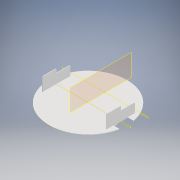
# Autodesk Inventor part: GonjaKonstrukcija_v.1.0
Saved by Autodesk Inventor 2020 (Build 240168000, 168)
## iProperties
Created: 2020-07-10
Part Number: GonjaKonstrukcija_v.1.0
Material: Generic
Document SubType Name: Modeling
Designer: Sičaja
Density: 1 g/cm^3
Appearance: Default
Author: Sičaja
Autodesk Inventor part; units mm, degrees
ref_plane "YZ Plane" through (0, 0, 0) normal (1, 0, 0) x (0, 1, 0)
ref_plane "XZ Plane" through (0, 0, 0) normal (0, 1, 0) x (-1, 0, 0)
ref_plane "XY Plane" through (0, 0, 0) normal (0, 0, 1) x (1, 0, 0)
sketch "Sketch1" plane through (0, 0, 0) normal (0, 1, 0) x (-1, 0, 0)
  circle A0 centre (0, 0) radius 75
  line L0 (20.1131, 19.7531) -> (28.825, 13.0373) projected
  line L1 (28.825, 13.0373) -> (16.004, -3.5946) projected
  line L2 (11.648, -0.2367) -> (16.004, -3.5946) projected
  line L3 (7.292, 3.1212) -> (11.648, -0.2367) projected
  line L4 (20.1131, 19.7531) -> (7.292, 3.1212) projected
  line L5 (4.487, 2.7582) -> (10.4269, -1.8207)
  line L6 (10.4269, -1.8207) -> (16.3669, -6.3997)
  line L7 (16.3669, -6.3997) -> (31.6301, 13.4002)
  line L8 (31.6301, 13.4002) -> (19.7502, 22.5581)
  line L9 (19.7502, 22.5581) -> (4.487, 2.7582)
  line L10 (16.3669, -6.3997) -> (31.6301, 13.4002)
  line L11 (19.7502, 22.5581) -> (4.487, 2.7582)
  line L12 (16.3669, -6.3997) -> (16.004, -3.5946)
  line L13 (28.825, 13.0373) -> (20.1131, 19.7531)
  line L14 (7.292, 3.1212) -> (16.004, -3.5946)
  line L15 (4.487, 2.7582) -> (16.3669, -6.3997)
  line L16 (32.309, 14.2809) -> (20.4291, 23.4389)
  line L17 (20.4291, 23.4389) -> (4.487, 2.7582)
  line L18 (16.3669, -6.3997) -> (32.309, 14.2809)
  line L19 (32.309, 14.2809) -> (16.3669, -6.3997)
  line L20 (4.487, 2.7582) -> (16.3669, -6.3997)
  line L21 (4.487, 2.7582) -> (20.4291, 23.4389)
  line L22 (32.309, 14.2809) -> (16.3669, -6.3997)
  line L23 (0, -32.563) -> (1, -32.563)
  line L24 (1, -32.563) -> (1, -33.063)
  line L25 (1, -33.063) -> (-1, -33.063)
  line L26 (-1, -33.063) -> (-1, -32.563)
  line L27 (-1, -32.563) -> (1, -32.563)
  dimension "d0" = 150
  dimension "d3" = 2
  dimension "d15" = 32.563
  dimension "d16" = 1
  dimension "d18" = 0.5
  dimension "d19" = 2
  dimension "d20" = 0.5
  constraints: 46 end point, 8 perpendicular, 4 collinear, 1 centre point, 1 coincident, 1 parallel, 1 vertical, 4 other
  measures "d0" diameter of A0
  measures "d3" distance between parallel lines of L4 L9
  measures "d15" distance of A0.centre L23.start
  measures "d16" distance of L23.start L23.end
  measures "d18" distance of L23.end L24.end
  measures "d19" distance of L24.end L25.end
  measures "d20" distance of L25.end L26.end
extrude "Extrusion1" add sketch "Sketch1" along normal blind 1 contours A0 | L0 L1 L2 L3 L4 | L9 L8 L7 L6 L5 | L17 L16 L18 L8 | L23 L24 L25 L26 L27
sketch "Sketch2" plane through (0, 0, 0) normal (0, -1, 0) x (1, 0, 0)
  circle A0 centre (0, 0) radius 75 projected
  line L0 (-20.7236, 20.5451) -> (-29.4356, 13.8293) projected
  line L1 (-29.4356, 13.8293) -> (-16.004, -3.5946) projected
  line L2 (-16.004, -3.5946) -> (-7.292, 3.1212) projected
  line L3 (-7.292, 3.1212) -> (-20.7236, 20.5451) projected
  line L4 (-4.487, 2.7582) -> (-16.3669, -6.3997)
  line L5 (-16.3669, -6.3997) -> (-32.2406, 14.1922)
  line L6 (-32.2406, 14.1922) -> (-20.3607, 23.3501)
  line L7 (-20.3607, 23.3501) -> (-4.487, 2.7582)
  dimension "d4" = 2
  constraints: 8 end point, 3 other
  measures "d4" distance between parallel lines of L2 L4
extrude "Extrusion2" cut sketch "Sketch2" against normal blind 1 contours L3 L2 L1 L0 | L4 L5 L6 L7
sketch "Sketch6" plane through (0, 1, 0) normal (0, 1, 0) x (1, 0, 0)
  line L0 (0, 32.563) -> (-1, 32.563)
  line L1 (-1, 32.563) -> (-1, 33.063)
  line L2 (-1, 33.063) -> (1, 33.063)
  line L3 (1, 33.063) -> (1, 32.563)
  line L4 (1, 32.563) -> (-1, 32.563)
  point P0 (0, 0)
  dimension "d21" = 32.563
  dimension "d22" = 1
  dimension "d23" = 0.5
  dimension "d24" = 2
  dimension "d25" = 0.5
  constraints: 10 end point, 2 perpendicular, 1 horizontal, 1 point on line
  measures "d21" distance of point (0, 0) L0.start
  measures "d22" distance of L0.start L0.end
  measures "d23" distance of L0.end L1.end
  measures "d24" distance of L1.end L2.end
  measures "d25" distance of L2.end L3.end
extrude "Extrusion4" add sketch "Sketch6" along normal blind 0.5
ref_plane "Work Plane1" through (0, 1, -32.563) normal (1, 0, 0) x (0, 0, -1)
ref_plane "Work Plane2" through (0.5, 1, -33.063) normal (0, 0, 1) x (1, 0, 0)
sketch "Sketch8" plane through (0, 1, 0) normal (0, 1, 0) x (1, 0, 0)
  line L0 (0.5, -0.5) -> (-0.5, -0.5)
  line L1 (-0.5, -0.5) -> (-0.5, 0.5)
  line L2 (-0.5, 0.5) -> (0.5, 0.5)
  line L3 (0.5, 0.5) -> (0.5, -0.5)
  line L4 (0.5, -0.5) -> (-0.5, 0.5) construction
  line L5 (-0.5, -0.5) -> (0.5, 0.5) construction
  point P0 (0, 0)
  dimension "d29" = 1
  dimension "d30" = 1
  constraints: 12 end point, 2 midpoint, 2 parallel, 1 horizontal, 1 perpendicular
  measures "d29" distance of L1.end L2.end
  measures "d30" distance of L0.end L1.end
extrude "Extrusion5" add sketch "Sketch8" along normal blind 0.5
ref_plane "Work Plane3" through (0.5, 1, 0) normal (0, 0, -1) x (-1, 0, 0)
sketch "Sketch9" plane through (0, 1, 0) normal (0, 1, 0) x (1, 0, 0)
  line L0 (-4.487, -2.7582) -> (-20.3607, -23.3501) projected
  line L1 (-16.3669, 6.3997) -> (-4.487, -2.7582) projected
  line L2 (-32.2406, -14.1922) -> (-16.3669, 6.3997) projected
  line L3 (-20.3607, -23.3501) -> (-32.2406, -14.1922) projected
  line L4 (0, -30.7284) -> (0, 15.3468)
  line L5 (4.487, -2.7582) -> (20.3607, -23.3501)
  line L6 (20.3607, -23.3501) -> (32.2406, -14.1922)
  line L7 (32.2406, -14.1922) -> (16.3669, 6.3997)
  line L8 (16.3669, 6.3997) -> (4.487, -2.7582)
  point P0 (0, 0)
  constraints: 10 end point, 4 symmetric about line, 1 vertical
extrude "Extrusion6" add sketch "Sketch9" against normal blind 1
sketch "Sketch10" plane through (0, 0, 0) normal (0, -1, 0) x (1, 0, 0)
  circle A0 centre (19.6481, -23.0808) radius 1.35 projected
  circle A1 centre (-15.7625, 22.8549) radius 1.35 projected
  circle A2 centre (23.0452, 52.7708) radius 1.35 projected
  circle A3 centre (58.4558, 6.8351) radius 1.35 projected
  circle A4 centre (-15.7625, 22.8549) radius 3 projected
  circle A5 centre (23.0452, 52.7708) radius 3 projected
  circle A6 centre (58.4558, 6.8351) radius 3 projected
  circle A7 centre (19.6481, -23.0808) radius 3 projected
  point P0 (0, 0)
extrude "Extrusion7" add sketch "Sketch10" along normal blind 3 contours A0 | A1 | A2 | A3 | A4 | A5 | A6 | A7
sketch "Sketch11" plane through (0, 0, 0) normal (0, -1, 0) x (1, 0, 0)
  line L0 (71.2588, -13.5) -> (62.3618, -13.5)
  line L1 (62.3618, -13.5) -> (62.3618, 13.5)
  line L2 (62.3618, 13.5) -> (71.2588, 13.5)
  circle A0 centre (0, 0) radius 75 projected
  line L3 (71.2588, 13.5) -> (73.775, 13.5)
  circle A1 centre (0, 0) radius 75 projected
  line L4 (71.2588, -13.5) -> (73.775, -13.5)
  line L5 (0, 23.2259) -> (0, -31.373)
  line L6 (-71.2588, -13.5) -> (-62.3618, -13.5)
  line L7 (-62.3618, -13.5) -> (-62.3618, 13.5)
  line L8 (-62.3618, 13.5) -> (-71.2588, 13.5)
  line L9 (-71.2588, 13.5) -> (-73.775, 13.5)
  line L10 (-71.2588, -13.5) -> (-73.775, -13.5)
  point P0 (-64.449, 0)
  dimension "d38" = 27
  constraints: 22 end point, 6 symmetric about line, 3 horizontal, 2 point on circle, 1 parallel, 1 perpendicular, 1 vertical
  measures "d38" distance of L0.end L1.end
extrude "Extrusion8" cut sketch "Sketch11" against normal blind 1 contours L0 L1 L2 L3 A0 L4 | A0 L9 L8 L7 L6 L10
sketch "Sketch17" plane through (0, 1, 0) normal (0, 1, 0) x (1, 0, 0)
  line L0 (-61.3618, 27.6098) -> (-62.3618, 27.6098)
  line L1 (-62.3618, 27.6098) -> (-62.3618, -26.3902)
  line L2 (-62.3618, -13.5) -> (-62.3618, 13.5) projected
  line L3 (-62.3618, -24.9796) -> (-62.3618, -27.3425)
  line L4 (-62.3618, -27.3425) -> (-61.3618, -27.3425)
  line L5 (-61.3618, -27.3425) -> (-62.3618, -27.3425)
  line L6 (-61.3618, 27.6098) -> (-61.3618, -26.3902)
  line L7 (-61.3618, 13.5) -> (-61.3618, -40.5) projected
  line L8 (-61.3618, -26.3902) -> (-62.3618, -26.3902)
  line L9 (-62.3618, 13.5) -> (-62.3618, -40.5) projected
  line L10 (-61.3618, -26.3902) -> (-62.3618, -26.3902)
  point P0 (0, 0)
  dimension "d53" = 54
  constraints: 16 end point, 2 collinear, 1 horizontal, 1 perpendicular
  measures "d53" distance of L0.start L6.end
extrude "Extrusion13" add sketch "Sketch17" along normal blind 25.5 contours L6 L8 L1 L0
sketch "Sketch18" plane through (-62.3618, 0, -13.5) normal (-1, 0, 0) x (0, 0, 1)
  line L0 (-14.1098, 1) -> (-14.1098, 26.5) projected
  line L1 (-14.1098, 18.7518) -> (12.4849, 18.7518)
  line L2 (12.4849, 18.7518) -> (12.4849, 26.5)
  line L3 (-14.1098, 26.5) -> (39.8902, 26.5) projected
  line L4 (12.4849, 26.5) -> (-14.1098, 26.5)
  point P0 (13.5, 0)
  constraints: 6 end point, 2 horizontal, 2 point on line, 1 perpendicular
extrude "Extrusion14" cut sketch "Sketch18" against normal blind 1
fillet "Fillet1" radius 2 3 edges at (-61.8618, 18.7518, -27.6098) (-61.8618, 26.5, -1.0151) (-61.8618, 26.5, 26.3902)
mirror "Mirror1" about plane through (0, 1, -32.563) normal (1, 0, 0) of "Extrusion13"
sketch "Sketch19" plane through (62.3618, 0, 13.5) normal (1, 0, 0) x (0, 0, -1)
  arc A0 (-10.8902, 26.5) -> (-12.8902, 24.5) centre (-10.8902, 24.5) ccw projected
  line L0 (39.1098, 18.7518) -> (14.5151, 18.7518) projected
  arc A1 (14.5151, 24.5) -> (12.5151, 26.5) centre (12.5151, 24.5) ccw projected
  line L1 (14.5151, 18.7518) -> (14.5151, 24.5) projected
  arc A2 (41.1098, 16.7518) -> (39.1098, 18.7518) centre (39.1098, 16.7518) ccw projected
  line L2 (41.1098, 1) -> (41.1098, 26.5) projected
  line L3 (37.079, 1) -> (18.1405, 1)
  line L4 (-12.8902, 1) -> (41.1098, 1) projected
  line L5 (-12.8902, 1) -> (-12.8902, 26.5) projected
  circle A3 centre (17.1098, 3) radius 1
  circle A4 centre (17.1098, 15.5) radius 1
  circle A5 centre (38.1098, 15.5) radius 1
  circle A6 centre (38.1098, 3) radius 1
  line L6 (41.1098, 26.5) -> (-12.8902, 26.5) projected
  line L7 (41.1098, 26.5) -> (-12.8902, 26.5)
  point P0 (13.5, 0)
  constraints: 4 centre point, 4 end point, 2 horizontal, 10 other
extrude "Extrusion15" cut sketch "Sketch19" against normal blind 1 contours A0 L5 L6 | L6 L2 A2 L0 L1 A1
body "Solid1"
